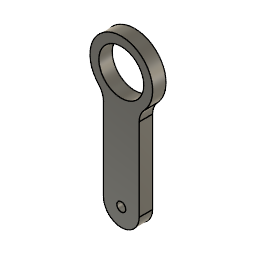
InputLink1 (Autodesk Fusion 360 design; units mm, degrees)
part number: 2026-02-01-16-20-52-191
Autodesk Fusion 360 part; units mm, degrees
sketch "Sketch1" plane through (0, 0, 0) normal (0, 1, 0) x (1, 0, 0)
  circle A0 centre (0, 0) radius 35
  circle A1 centre (0, 0) radius 25
  line L0 (-20, 28.7228) -> (20, 28.7228)
  dimension "d1" = 70
  dimension "d2" = 50
  dimension "d3" = 40
  constraint coincident A0.centre A1.centre
  constraint concentric A0 A1
  constraint coincident A0 L0.start
  constraint coincident A0 L0.end
  constraint horizontal L0
  measures "d1" diameter of A0
  measures "d2" diameter of A1
  measures "d3" distance of L0.start L0.end
extrude "Extrude1" add sketch "Sketch1" along normal mid plane 15
ref_plane "WorkPlane1" through (0, 0, -50) normal (0, 0, 1) x (1, 0, 0)
sketch "Sketch2" plane through (0, 0, -50) normal (0, 0, 1) x (1, 0, 0)
  line L0 (20, 7.5) -> (-20, 7.5)
  line L1 (-20, 7.5) -> (-20, -7.5)
  line L2 (-20, -7.5) -> (20, -7.5)
  line L3 (20, -7.5) -> (20, 7.5)
  line L4 (20, 7.5) -> (-20, -7.5) construction
  line L5 (-20, 7.5) -> (20, -7.5) construction
  dimension "d7" = 40
  dimension "d8" = 15
  constraint horizontal L0
  constraint perpendicular L0 L1
  constraint parallel L0 L2
  constraint parallel L1 L3
  constraint coincident L4 origin
  constraint coincident L5 origin
  measures "d7" distance of L1.end L2.end
  measures "d8" distance of L0.end L1.end
extrude "Extrude2" add sketch "Sketch2" along normal blind 23 and the other way blind 100
fillet "Fillet1" radius 20 2 edges at (20, 0, -28.7228) (-20, 0, -28.7228)
fillet "Fillet1" radius 20 2 edges at (20, 0, -150) (-20, 0, -150)
sketch "Sketch3" plane through (0, -7.5, 0) normal (0, -1, 0) x (1, 0, 0)
  circle A0 centre (0, 0) radius 25
  arc A1 (-20, -130) -> (20, -130) centre (0, -130) ccw
  line L0 (20, -130) -> (20, -37.7492)
  arc A2 (25.4545, -24.0222) -> (20, -37.7492) centre (40, -37.7492) ccw
  arc A3 (25.4545, -24.0222) -> (-25.4545, -24.0222) centre (0, 0) ccw
  arc A4 (-20, -37.7492) -> (-25.4545, -24.0222) centre (-40, -37.7492) ccw
  line L1 (-20, -37.7492) -> (-20, -130)
  circle A5 centre (0, -130) radius 5
  dimension "d17" = 10
  constraint concentric A1 A5
  measures "d17" diameter of A5
extrude "Extrude3" cut sketch "Sketch3" against normal through all contours A5
